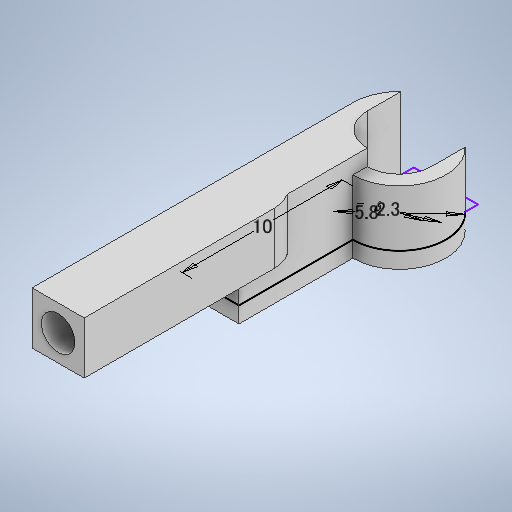
# Autodesk Inventor part: srod1.5right
Saved by Autodesk Inventor 2025 (Build 290162000, 162)
## iProperties
Created: 2024-07-29
Part Number: srod1.5right
Material: 一般
Document SubType Name: Modeling
Designer: Saigusa
Density: 1 g/cm^3
Appearance: 既定
Author: Saigusa
Autodesk Inventor part; units mm, degrees
ref_plane "YZ Plane" through (0, 0, 0) normal (1, 0, 0) x (0, 1, 0)
ref_plane "XZ Plane" through (0, 0, 0) normal (0, 1, 0) x (-1, 0, 0)
ref_plane "XY Plane" through (0, 0, 0) normal (0, 0, 1) x (1, 0, 0)
sketch "スケッチ1" plane through (0, 0, 0) normal (0, 1, 0) x (-1, 0, 0)
  circle A0 centre (0, 0) radius 1.15
  circle A1 centre (0, 0) radius 2
  circle A2 centre (0, 0) radius 2.9
  line L0 (-2, 0) -> (2, 0)
  line L1 (2, 0) -> (2, -2.9)
  line L2 (2, -2.9) -> (-2, -2.9)
  line L3 (-2, -2.9) -> (-2, 0)
  line L4 (0, 0) -> (0, 2.9)
  line L5 (0, 0) -> (2.9, 0)
  line L6 (2.9, 0) -> (2.9, 10)
  line L7 (2.9, 10) -> (0, 10)
  line L8 (0, 10) -> (0, 0)
  point P0 (0, 2)
  point P1 (2, -2.1)
  point P2 (-2, -2.1)
  dimension "d1" = 4
  dimension "d2" = 5.8
  dimension "d0" = 2.3
  dimension "d3" = 10
  constraints: 18 end point, 4 parallel, 3 coincident, 2 horizontal, 2 perpendicular, 1 centre point, 1 vertical, 6 other
  measures "d0" diameter of A0
  measures "d3" distance of L6.end L5.end
extrude "押し出し1" add sketch "スケッチ1" along normal blind 4.5 contours L5 A2 L1 | A1 L4 A2 L5 | A2 L8 L7 L6
extrude "押し出し2" add sketch "スケッチ1" along normal blind 3.5 contours A1 L3 A2 L4
extrude "押し出し3" add sketch "スケッチ1" against normal blind 1 contours L0 A1 A0 | A0 L4 A1 L0 | A0 L0 A1 L4 | L1 A2 L3 A1 | L5 A2 L1 | A1 L4 A2 L5 | A1 L3 A2 L4 | A2 L8 L7 L6
sketch "スケッチ2" plane through (-2.9, 4.5, 10) normal (0, 0, 1) x (1, 0, 0)
  line L0 (2.9, -4.5) -> (1.4, -4.5)
  line L1 (1.4, -4.5) -> (1.4, -4)
  line L2 (1.4, -4) -> (2.9, -4)
  line L3 (2.9, -4) -> (2.9, -4.5)
  dimension "d10" = 1.5
  dimension "d11" = 0.5
  constraints: 8 end point, 2 parallel, 1 horizontal, 1 perpendicular
  measures "d10" distance of L1.end L2.end
  measures "d11" distance of L0.end L1.end
hole "穴1" at (-1.5, 0.5, 10) direction (0, 0, -1) diameter 1 end through all
sketch "スケッチ3" plane through (-2.9, 4.5, 10) normal (0, 0, 1) x (1, 0, 0)
  line L0 (0.9, 0) -> (0, 0) projected
  line L1 (0, 0) -> (4, 0)
  line L2 (4, 0) -> (4, -4)
  line L3 (4, -4) -> (0, -4)
  line L4 (0, -4) -> (0, 0)
  line L5 (0, 0) -> (3.25, 0)
  line L6 (3.25, 0) -> (3.25, -3.25)
  line L7 (3.25, -3.25) -> (0, -3.25)
  line L8 (0, -3.25) -> (0, 0)
  line L9 (0, 0) -> (1.625, 0)
  line L10 (1.625, 0) -> (1.625, -1.625)
  line L11 (1.625, -1.625) -> (0, -1.625)
  line L12 (0, -1.625) -> (0, 0)
  point P0 (2.9, -4.5)
  dimension "d19" = 4
  dimension "d20" = 4
  dimension "d21" = 3.25
  dimension "d22" = 3.25
  constraints: 24 end point, 6 parallel, 3 horizontal, 3 perpendicular
  measures "d19" distance of L2.end L3.end
  measures "d20" distance of L1.end L2.end
  measures "d21" distance of L6.end L7.end
  measures "d22" distance of L5.end L6.end
extrude "押し出し4" add sketch "スケッチ3" along normal blind 10 and the other way blind 3 contours L1 L10 L11 L4 L0 | L1 L6 L7 L4 L11 L10
fillet "フィレット1" radius 2 1 edges at (0.35, 2.875, 7)
sketch "スケッチ4" plane through (-2.9, 4.5, 20) normal (0, 0, 1) x (1, 0, 0)
  line L0 (0.9, 0) -> (0, 0) projected
  line L1 (0, 0) -> (1.625, 0)
  line L2 (1.625, 0) -> (1.625, -1.625)
  line L3 (1.625, -1.625) -> (0, -1.625)
  line L4 (0, -1.625) -> (0, 0)
  circle A0 centre (1.625, -1.625) radius 1.05
  point P0 (2.9, -4.5)
  dimension "d28" = 1.625
  dimension "d29" = 1.625
  dimension "d30" = 2.1
  constraints: 8 end point, 2 parallel, 1 centre point, 1 coincident, 1 horizontal, 1 perpendicular
  measures "d28" distance of L2.end L3.end
  measures "d29" distance of L1.end L2.end
  measures "d30" diameter of A0
extrude "押し出し5" cut sketch "スケッチ4" against normal blind 11 contours A0 L3 L2 | L2 L3 A0
